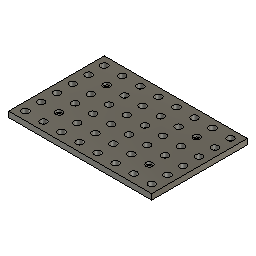
48_vial_plate_retainerLid v2 (Autodesk Fusion 360 design; units mm, degrees)
Autodesk Fusion 360 part; units mm, degrees
note: some values were not read from the file. Set by a fixed rule: the direction of a hole.
sketch "Sketch1" plane through (0, 0, 0) normal (0, 0, 1) x (1, 0, 0)
  line L0 (0, 0) -> (127.76, 0)
  line L1 (127.76, 0) -> (127.76, -85.48)
  line L2 (127.76, -85.48) -> (0, -85.48)
  line L3 (0, -85.48) -> (0, 0)
  dimension "d1" = 127.76
  dimension "d2" = 85.48
  constraint horizontal L0
  constraint vertical L1
  constraint horizontal L2
  constraint vertical L3
  constraint coincident L0.start L3.end
  measures "d1" distance of L0.start L0.end
  measures "d2" distance of L0.start L2.end
extrude "Extrude1" add sketch "Sketch1" along normal blind 18
move_face "OffsetFaces1" offset -13 1 faces at (42.5867, -28.4933, 0)
sketch "Sketch2" plane through (0, 0, 13) normal (0, 0, 1) x (-1, 0, 0)
  line L0 (0, 85.48) -> (-127.76, 85.48)
  line L1 (-127.76, 85.48) -> (-127.76, 0)
  line L2 (-127.76, 0) -> (0, 0)
  line L3 (0, 0) -> (0, 85.48)
  line L4 (0, 85.48) -> (-127.76, 85.48)
  line L5 (-127.76, 85.48) -> (-127.76, 0)
  line L6 (-127.76, 0) -> (0, 0)
  line L7 (0, 0) -> (0, 85.48)
  line L8 (-127.76, 85.48) -> (0, 85.48)
  line L9 (0, 85.48) -> (0, 0)
  line L10 (0, 0) -> (-127.76, 0)
  line L11 (-127.76, 0) -> (-127.76, 85.48)
  line L12 (-127.76, 85.48) -> (0, 85.48)
  line L13 (0, 85.48) -> (0, 0)
  line L14 (0, 0) -> (-127.76, 0)
  line L15 (-127.76, 0) -> (-127.76, 85.48)
  point P0 (-7.5, 7.5)
  point P1 (-23.6086, 7.5)
  point P2 (-39.7171, 7.5)
  point P3 (-55.8257, 7.5)
  point P4 (-71.9343, 7.5)
  point P5 (-88.0429, 7.5)
  point P6 (-104.1514, 7.5)
  point P7 (-120.26, 7.5)
  point P8 (-7.5, 21.596)
  point P9 (-23.6086, 21.596)
  point P10 (-39.7171, 21.596)
  point P11 (-55.8257, 21.596)
  point P12 (-71.9343, 21.596)
  point P13 (-88.0429, 21.596)
  point P14 (-104.1514, 21.596)
  point P15 (-120.26, 21.596)
  point P16 (-7.5, 35.692)
  point P17 (-23.6086, 35.692)
  point P18 (-39.7171, 35.692)
  point P19 (-55.8257, 35.692)
  point P20 (-71.9343, 35.692)
  point P21 (-88.0429, 35.692)
  point P22 (-104.1514, 35.692)
  point P23 (-120.26, 35.692)
  point P24 (-7.5, 49.788)
  point P25 (-23.6086, 49.788)
  point P26 (-39.7171, 49.788)
  point P27 (-55.8257, 49.788)
  point P28 (-71.9343, 49.788)
  point P29 (-88.0429, 49.788)
  point P30 (-104.1514, 49.788)
  point P31 (-120.26, 49.788)
  point P32 (-7.5, 63.884)
  point P33 (-23.6086, 63.884)
  point P34 (-39.7171, 63.884)
  point P35 (-55.8257, 63.884)
  point P36 (-71.9343, 63.884)
  point P37 (-88.0429, 63.884)
  point P38 (-104.1514, 63.884)
  point P39 (-120.26, 63.884)
  point P40 (-7.5, 77.98)
  point P41 (-23.6086, 77.98)
  point P42 (-39.7171, 77.98)
  point P43 (-55.8257, 77.98)
  point P44 (-71.9343, 77.98)
  point P45 (-88.0429, 77.98)
  point P46 (-104.1514, 77.98)
  point P47 (-120.26, 77.98)
  dimension "d7" = -16.1086
  dimension "d8" = 14.096
hole "Hole1" at (7.5, -7.5, 13) at (23.6086, -7.5, 13) at (39.7171, -7.5, 13) at (55.8257, -7.5, 13) at (71.9343, -7.5, 13) at (88.0429, -7.5, 13) at (104.1514, -7.5, 13) at (120.26, -7.5, 13) at (7.5, -21.596, 13) at (39.7171, -21.596, 13) at (55.8257, -21.596, 13) at (71.9343, -21.596, 13) at (88.0429, -21.596, 13) at (120.26, -21.596, 13) at (120.26, -63.884, 13) at (7.5, -77.98, 13) at (7.5, -35.692, 13) at (7.5, -49.788, 13) at (7.5, -63.884, 13) at (120.26, -35.692, 13) at (55.8257, -35.692, 13) at (39.7171, -77.98, 13) at (88.0429, -35.692, 13) at (55.8257, -77.98, 13) at (23.6086, -35.692, 13) at (88.0429, -63.884, 13) at (39.7171, -49.788, 13) at (71.9343, -35.692, 13) at (120.26, -49.788, 13) at (88.0429, -77.98, 13) at (104.1514, -35.692, 13) at (88.0429, -49.788, 13) at (104.1514, -49.788, 13) at (120.26, -77.98, 13) at (71.9343, -77.98, 13) at (71.9343, -49.788, 13) at (104.1514, -77.98, 13) at (39.7171, -63.884, 13) at (23.6086, -49.788, 13) at (71.9343, -63.884, 13) at (55.8257, -49.788, 13) at (23.6086, -77.98, 13) at (39.7171, -35.692, 13) at (55.8257, -63.884, 13) direction (0, 0, 1) diameter 6 depth 13 tip angle 180 counterbore diameter 12 counterbore depth 1
sketch "Sketch6" plane through (0, 0, 18) normal (0, 0, 1) x (-1, 0, 0)
  line L0 (0, 85.48) -> (-127.76, 85.48)
  line L1 (-127.76, 85.48) -> (-127.76, 0)
  line L2 (-127.76, 0) -> (0, 0)
  line L3 (0, 0) -> (0, 85.48)
  circle A0 centre (-39.7171, 35.692) radius 3
  circle A1 centre (-55.8257, 49.788) radius 3
  circle A2 centre (-23.6086, 49.788) radius 3
  circle A3 centre (-104.1514, 77.98) radius 3
  circle A4 centre (-71.9343, 77.98) radius 3
  circle A5 centre (-104.1514, 49.788) radius 3
  circle A6 centre (-104.1514, 35.692) radius 3
  circle A7 centre (-120.26, 49.788) radius 3
  circle A8 centre (-39.7171, 49.788) radius 3
  circle A9 centre (-23.6086, 35.692) radius 3
  circle A10 centre (-88.0429, 35.692) radius 3
  circle A11 centre (-55.8257, 35.692) radius 3
  circle A12 centre (-7.5, 63.884) radius 3
  circle A13 centre (-7.5, 35.692) radius 3
  circle A14 centre (-120.26, 63.884) radius 3
  circle A15 centre (-88.0429, 21.596) radius 3
  circle A16 centre (-55.8257, 21.596) radius 3
  circle A17 centre (-7.5, 21.596) radius 3
  circle A18 centre (-104.1514, 7.5) radius 3
  circle A19 centre (-71.9343, 7.5) radius 3
  circle A20 centre (-39.7171, 7.5) radius 3
  circle A21 centre (-7.5, 7.5) radius 3
  circle A22 centre (-23.6086, 7.5) radius 3
  circle A23 centre (-55.8257, 7.5) radius 3
  circle A24 centre (-88.0429, 7.5) radius 3
  circle A25 centre (-120.26, 7.5) radius 3
  circle A26 centre (-39.7171, 21.596) radius 3
  circle A27 centre (-71.9343, 21.596) radius 3
  circle A28 centre (-120.26, 21.596) radius 3
  circle A29 centre (-7.5, 77.98) radius 3
  circle A30 centre (-7.5, 49.788) radius 3
  circle A31 centre (-120.26, 35.692) radius 3
  circle A32 centre (-39.7171, 77.98) radius 3
  circle A33 centre (-55.8257, 77.98) radius 3
  circle A34 centre (-88.0429, 63.884) radius 3
  circle A35 centre (-71.9343, 35.692) radius 3
  circle A36 centre (-88.0429, 77.98) radius 3
  circle A37 centre (-88.0429, 49.788) radius 3
  circle A38 centre (-120.26, 77.98) radius 3
  circle A39 centre (-71.9343, 49.788) radius 3
  circle A40 centre (-39.7171, 63.884) radius 3
  circle A41 centre (-71.9343, 63.884) radius 3
  circle A42 centre (-23.6086, 77.98) radius 3
  circle A43 centre (-55.8257, 63.884) radius 3
  point P0 (-104.1514, 63.884)
  point P1 (-104.1514, 21.596)
  point P2 (-23.6086, 21.596)
  point P3 (-23.6086, 63.884)
  constraint vertical P0 P1
  constraint horizontal P1 P2
  constraint vertical P2 P3
hole "Hole2" at (104.1514, -63.884, 18) at (104.1514, -21.596, 18) at (23.6086, -63.884, 18) at (23.6086, -21.596, 18) direction (0, 0, -1) diameter 3.4 depth 20 tip angle 180 counterbore diameter 6 counterbore depth 2
